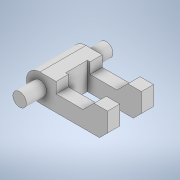
# Autodesk Inventor part: 10-2
Saved by Autodesk Inventor 2022 (Build 260153000, 153)
## iProperties
Created: 2021-09-12
Part Number: 10-2
Material: 일반
Document SubType Name: Modeling
Designer: 서울공업고등학교
Density: 1 g/cm^3
Appearance: 기본값
Author: 서울공업고등학교
Autodesk Inventor part; units mm, degrees
ref_plane "YZ Plane" through (0, 0, 0) normal (1, 0, 0) x (0, 1, 0)
ref_plane "XZ Plane" through (0, 0, 0) normal (0, 1, 0) x (-1, 0, 0)
ref_plane "XY Plane" through (0, 0, 0) normal (0, 0, 1) x (1, 0, 0)
sketch "스케치1" plane through (0, 0, 0) normal (0, 0, 1) x (1, 0, 0)
  circle A0 centre (0, 0) radius 2.5
  circle A1 centre (0, 0) radius 5
  line L0 (0, -5) -> (25, -5)
  line L1 (25, -5) -> (25, 5)
  line L2 (25, 5) -> (20, 5)
  line L3 (20, 5) -> (16, 1)
  line L4 (16, 1) -> (6, 1)
  line L5 (6, 1) -> (6, 5)
  line L6 (6, 5) -> (0, 5)
  dimension "d0" = 5
  dimension "d1" = 10
  dimension "d2" = 25
  dimension "d3" = 10
  dimension "d4" = 90
  dimension "d5" = 5
  dimension "d6" = 90
  dimension "d7" = 10
  dimension "d8" = 4
  dimension "d9" = 4
  constraints: 14 end point, 3 perpendicular, 2 centre point, 2 coincident, 2 parallel, 2 point on circle, 1 horizontal, 1 point on line, 1 tangent
  measures "d0" diameter of A0
  measures "d1" diameter of A1
  measures "d2" distance of L0.start L0.end
  measures "d3" distance of L0.end L1.end
  measures "d4" angle of L1 L0
  measures "d5" distance of L1.end L2.end
  measures "d6" angle of L2 L1
  measures "d7" distance of L3.end L4.end
  measures "d8" distance of L4.end L5.end
  measures "d9" horizontal distance of L3.end L2.end
extrude "돌출1" add sketch "스케치1" along normal mid plane 17
extrude "돌출2" add sketch "스케치1" along normal mid plane 32 contours A0
sketch "스케치2" plane through (0, 0, 0) normal (0, 0, 1) x (1, 0, 0)
  line L0 (5, 11.5318) -> (29.4408, 11.5318)
  line L1 (29.4408, 11.5318) -> (29.4408, -9.0869)
  line L2 (29.4408, -9.0869) -> (5, -9.0869)
  line L3 (5, -9.0869) -> (5, 11.5318)
  line L4 (25, 5) -> (25, -5) projected
  point P0 (0, 0)
  dimension "d14" = 20
  constraints: 8 end point, 2 parallel, 1 horizontal, 1 perpendicular
  measures "d14" distance between parallel lines of L3 L4
extrude "돌출3" cut sketch "스케치2" along normal mid plane 8
chamfer "모따기1" distance 3 angle 45 2 edges at (25, -5, 6.25) (25, -5, -6.25)
